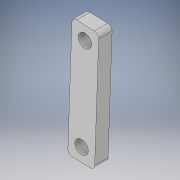
# Autodesk Inventor part: Connector Boi
Saved by Autodesk Inventor 2019 (Build 230136000, 136)
## iProperties
Created: 2019-06-11
Part Number: Connector Boi
Material: Generic
Document SubType Name: Modeling
Designer: Cole
Density: 1 g/cm^3
Appearance: Default
Author: Cole
Autodesk Inventor part; units mm, degrees
ref_plane "YZ Plane" through (0, 0, 0) normal (1, 0, 0) x (0, 1, 0)
ref_plane "XZ Plane" through (0, 0, 0) normal (0, 1, 0) x (-1, 0, 0)
ref_plane "XY Plane" through (0, 0, 0) normal (0, 0, 1) x (1, 0, 0)
sketch "Sketch1" plane through (0, 0, 0) normal (0, 0, 1) x (1, 0, 0)
  line L0 (-1.0667, -1.8887) -> (-0.1724, 23.0976)
  line L1 (0.8627, 24.0612) -> (4.8545, 23.9183)
  line L2 (5.8181, 22.8832) -> (4.9238, -2.1031)
  line L3 (3.8887, -3.0667) -> (-0.1031, -2.9238)
  circle A0 centre (2, 0) radius 1.4986
  circle A1 centre (2.7514, 20.9945) radius 1.4986
  circle A2 centre (2.7514, 20.9945) radius 1.4986 projected
  circle A3 centre (2, 0) radius 1.4986 projected
  arc A4 (-1.0667, -1.8887) -> (-0.1031, -2.9238) centre (-0.0674, -1.9245) ccw
  arc A5 (3.8887, -3.0667) -> (4.9238, -2.1031) centre (3.9245, -2.0674) ccw
  arc A6 (5.8181, 22.8832) -> (4.8545, 23.9183) centre (4.8188, 22.919) ccw
  arc A7 (0.8627, 24.0612) -> (-0.1724, 23.0976) centre (0.8269, 23.0619) ccw
  point P0 (0, 0)
  dimension "d0" = 5.9944
  dimension "d1" = 2.9972
  dimension "d2" = 2.9972
  dimension "d3" = 2.9972
  dimension "d4" = 2.9972
  dimension "d6" = 2.9972
  dimension "d7" = 2.9972
  dimension "d8" = 1
  constraints: 8 end point, 8 point on circle, 8 tangent, 6 centre point, 3 equal radius, 3 perpendicular, 2 coincident
  measures "d0" distance between parallel lines of L0 L2
  measures "d1" diameter of A1
  measures "d2" diameter of A0
  measures "d3" distance from line of L0 A0.centre
  measures "d4" distance from line of A0.centre L3
  measures "d6" distance from line of L0 A1.centre
  measures "d7" distance from line of L1 A1.centre
  measures "d8" radius of A4
extrude "Extrusion1" add sketch "Sketch1" along normal blind 3
equation "\"d2\" = d1"
equation "\"d3\" = d2"
equation "\"d4\" = d2"
equation "\"d6\" = d1"
body "Solid1"
